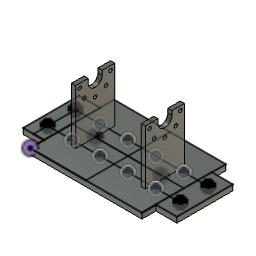
final hinge (Autodesk Fusion 360 design; units mm, degrees)
Autodesk Fusion 360 part; units mm, degrees
sketch "스케치1" plane through (0, 0, 0) normal (0, 0, 1) x (1, 0, 0)
  line L0 (0, 0) -> (80, 0)
  line L1 (80, 0) -> (80, 60)
  line L2 (80, 60) -> (0, 60)
  line L3 (0, 60) -> (0, 0)
  line L4 (0, 0) -> (0, 10)
  line L5 (0, 10) -> (-15, 10)
  line L6 (-15, 10) -> (-15, 50)
  line L7 (-15, 50) -> (0, 50)
  line L8 (0, 50) -> (0, 10)
  line L9 (80, 0) -> (80, 10)
  line L10 (80, 10) -> (95, 10)
  line L11 (95, 10) -> (95, 50)
  line L12 (95, 50) -> (80, 50)
  line L13 (80, 50) -> (80, 10)
  line L14 (0, 10) -> (-7.5, 10)
  line L15 (0, 0) -> (0, 30)
  line L16 (-7.5, 10) -> (-7.5, 20)
  line L17 (-7.5, 20) -> (-7.5, 40)
  circle A0 centre (-7.5, 40) radius 1.5
  circle A1 centre (-7.5, 20) radius 1.5
  line L18 (-7.5, 40) -> (87.5, 40)
  line L19 (-7.5, 20) -> (87.5, 20)
  circle A2 centre (10, 40) radius 1.5
  circle A3 centre (30, 40) radius 1.5
  circle A4 centre (50, 40) radius 1.5
  circle A5 centre (70, 40) radius 1.5
  circle A6 centre (87.5, 40) radius 1.5
  circle A7 centre (10, 20) radius 1.5
  circle A8 centre (30, 20) radius 1.5
  circle A9 centre (50, 20) radius 1.5
  circle A10 centre (70, 20) radius 1.5
  circle A11 centre (87.5, 20) radius 1.5
  line L20 (0, 0) -> (40, 0)
  line L21 (40, 0) -> (40, 60)
  line L22 (0, 30) -> (80, 30)
  line L23 (40, 30) -> (16.5, 30)
  line L24 (40, 30) -> (63.5, 30)
  dimension "d1" = 80
  dimension "d2" = 60
  dimension "d3" = 10
  dimension "d4" = 15
  dimension "d5" = 40
  dimension "d6" = 10
  dimension "d7" = 15
  dimension "d8" = 40
  dimension "d10" = 10
  dimension "d11" = 20
  dimension "d12" = 3
  dimension "d13" = 3
  dimension "d14" = 95
  dimension "d15" = 95
  dimension "d16" = 3
  dimension "d17" = 3
  dimension "d18" = 3
  dimension "d19" = 3
  dimension "d20" = 3
  dimension "d21" = 3
  dimension "d22" = 3
  dimension "d23" = 3
  dimension "d24" = 3
  dimension "d25" = 3
  dimension "d45" = 23.5
  dimension "d46" = 23.5
  constraint horizontal L0
  constraint vertical L1
  constraint horizontal L2
  constraint vertical L3
  constraint coincident L0.start L3.end
  constraint perpendicular L0 L4
  constraint horizontal L5
  constraint vertical L6
  constraint horizontal L7
  constraint vertical L8
  constraint perpendicular L0 L9
  constraint horizontal L10
  constraint vertical L11
  constraint horizontal L12
  constraint vertical L13
  constraint midpoint L5 L14.end
  constraint midpoint L8 L15.end
  constraint perpendicular L5 L16
  constraint perpendicular L14 L17
  constraint coincident L17.end A0.centre
  constraint coincident L16.end L17.start
  constraint perpendicular L1 L18
  constraint perpendicular L11 L19
  constraint coincident L18 A2.centre
  constraint coincident L18 A3.centre
  constraint coincident L18 A4.centre
  constraint coincident L18 A5.centre
  constraint coincident L18.end A6.centre
  constraint coincident L19 A7.centre
  constraint coincident L19 A8.centre
  constraint coincident L19 A9.centre
  constraint coincident L19 A10.centre
  constraint coincident L19.end A11.centre
  constraint midpoint L0 L20.end
  constraint midpoint L2 L21.end
  constraint midpoint L1 L22.end
  constraint midpoint L22 L23.start
  constraint perpendicular L21 L23
  constraint perpendicular L21 L24
  measures "d1" distance of L0.start L0.end
  measures "d2" distance of L0.start L2.end
  measures "d3" distance of L0.start L4.end
  measures "d4" distance of L4.end L5.end
  measures "d5" distance of L4.end L7.end
  measures "d6" distance of L0.end L9.end
  measures "d7" distance of L9.end L10.end
  measures "d8" distance of L9.end L12.end
  measures "d10" distance of L14.end L16.end
  measures "d11" distance of L16.end L17.end
  measures "d12" diameter of A0
  measures "d13" diameter of A1
  measures "d14" distance of L17.end L18.end
  measures "d15" distance of L16.end L19.end
  measures "d16" diameter of A2
  measures "d17" diameter of A3
  measures "d18" diameter of A4
  measures "d19" diameter of A5
  measures "d20" diameter of A6
  measures "d21" diameter of A7
  measures "d22" diameter of A8
  measures "d23" diameter of A9
  measures "d24" diameter of A10
  measures "d25" diameter of A11
  measures "d45" distance of L23.start L23.end
  measures "d46" distance of L23.start L24.end
sketch "스케치2" plane through (0, 0, 0) normal (1, 0, 0) x (0, 1, 0)
  line L0 (0, 0) -> (16, 0)
  line L1 (16, 0) -> (44, 0)
  line L2 (44, 0) -> (44, 39)
  line L3 (16, 39) -> (16, 0)
  line L4 (16, 39) -> (25, 39)
  line L5 (16, 39) -> (16, 36)
  line L6 (16, 36) -> (25, 36)
  line L7 (16, 36) -> (25, 36)
  line L8 (35, 36) -> (35, 39)
  line L9 (25, 39) -> (25, 36)
  arc A0 (25, 36) -> (35, 36) centre (30, 36) ccw
  line L10 (44, 39) -> (35, 39)
  line L11 (25, 39) -> (16, 39)
  line L12 (26.4645, 32.4645) -> (22.2218, 28.2218)
  line L13 (30, 36) -> (41, 36) construction
  line L14 (33.5355, 32.4645) -> (37.7782, 28.2218)
  line L15 (30, 36) -> (41, 36) construction
  line L16 (30, 31) -> (30, 25)
  line L17 (30, 36) -> (30, 25)
  arc A1 (19, 36) -> (41, 36) centre (30, 36) ccw
  circle A2 centre (19, 36) radius 1.25
  circle A3 centre (22.2218, 28.2218) radius 1.25
  circle A4 centre (30, 25) radius 1.25
  circle A5 centre (37.7782, 28.2218) radius 1.25
  circle A6 centre (41, 36) radius 1.25
  dimension "d26" = 16
  dimension "d27" = 28
  dimension "d28" = 39
  dimension "d29" = 3
  dimension "d30" = 9
  dimension "d31" = 10
  dimension "d32" = 3
  dimension "d33" = 10
  dimension "d34" = 22
  dimension "d35" = 135
  dimension "d36" = 11
  dimension "d37" = 45
  dimension "d38" = 2.5
  dimension "d39" = 2.5
  dimension "d40" = 2.5
  dimension "d41" = 2.5
  dimension "d42" = 2.5
  constraint coincident L0.start origin
  constraint horizontal L0
  constraint horizontal L1
  constraint vertical L2
  constraint horizontal L10
  constraint vertical L3
  constraint perpendicular L5 L10
  constraint perpendicular L3 L6
  constraint perpendicular L5 L7
  constraint vertical L8
  constraint vertical L9
  constraint collinear L10 L11
  constraint concentric A0 A1
  constraint horizontal L13
  constraint coincident A0.centre L13.start
  constraint horizontal L15
  constraint coincident L16.end A1
  constraint vertical L16
  constraint coincident A0 L14.start
  constraint coincident A0 L12.start
  constraint coincident A0 L16.start
  constraint coincident L6 A1.start
  constraint coincident A1.start A2.centre
  constraint coincident L12.end A3.centre
  constraint coincident L16.end L17.end
  constraint coincident L14.end A5.centre
  constraint coincident L13.end L15.end
  measures "d26" distance of L0.start L0.end
  measures "d27" distance of L0.end L1.end
  measures "d28" distance of L0.end L3.start
  measures "d29" distance of L3.start L5.end
  measures "d30" distance of L5.end L6.end
  measures "d31" distance of L6.end L8.start
  measures "d32" distance of L6.end L4.end
  measures "d33" diameter of A0
  measures "d34" diameter of A1
  measures "d35" angle of L12 L13
  measures "d36" distance of A0.centre L12.end
  measures "d37" angle of L14 L15
  measures "d38" diameter of A2
  measures "d39" diameter of A3
  measures "d40" diameter of A4
  measures "d41" diameter of A5
  measures "d42" diameter of A6
extrude "돌출1" add sketch "스케치1" against normal blind 4 contours L0 L3 L4 L8 L15 L19 A7 A8 L20 L21 | L0 L1 L9 L13 L19 A9 A10 L21 | L3 L5 L8 L14 L15 L16 A1 L19 | L1 L13 L19 A9 A10 L21 L22 L24 | L3 L8 L15 L19 A7 A8 L21 L22 L23 | L3 L8 L15 L17 A0 A1 L18 L19 | L3 L5 L6 L7 L8 L16 L17 A0 A1 L18 | L1 L10 L11 L12 L13 | L3 L8 L18 A2 A3 L21 L22 L23 | L1 L13 L18 A4 A5 L21 L22 L24 | L1 L2 L13 L18 A4 A5 L21 | L2 L3 L8 L18 A2 A3 L21 makes body 1
extrude "돌출2" add sketch "스케치2" against normal blind 3 separate body contours L1 L2 L3 L6 L7 L8 A0 L10 L14 A1 A2 A3 A4 A5 | L3 L4 L5 L6 L7 L9 L11 A2 | L6 L7 A0 L12 A1 A2 A3 | A0 L14 L16 L17 A1 A4 A5 | A0 L12 L16 L17 A1 A3 A4 makes body 2
move_body "이동1" bodies 2 to x (1, 0, 0) y (0, 1, 0) z (0, 0, 1) at (16.5, 0, 0)
copy_body "CopyPasteBodies1" bodies 2 makes body 3
move_body "이동2" bodies 3 to x (1, 0, 0) y (0, 1, 0) z (0, 0, 1) at (50, 0, 0)
named bodies: "전면판", "옆판1", "옆판2"
